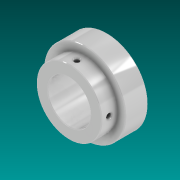
# Autodesk Inventor part: bovenkantGearbox
Saved by Autodesk Inventor 2020.2 (Build 242310000, 310)
## iProperties
Created: 2020-05-14
Part Number: bovenkantGearbox
Material: Aluminum 6061
Document SubType Name: Modeling
Designer: Svend
Density: 2.7 g/cm^3
Appearance: Aluminum - Polished
Author: Svend
Autodesk Inventor part; units mm, degrees
sketch "Sketch1" plane through (0, 0, 0) normal (0, 0, 1) x (1, 0, 0)
  circle A0 centre (0, 0) radius 21
  circle A1 centre (0, 0) radius 12.5
  circle A2 centre (0, 0) radius 11
  point P0 (18, 0)
  point P1 (0, 18)
  point P2 (-18, 0)
  point P3 (0, -18)
  dimension "d0" = 42
  dimension "d1" = 25
  dimension "d2" = 22
  dimension "d3" = 18
  dimension "d6" = 360
  constraints: 6 coincident, 3 centre point, 1 horizontal alignment, 7 other
  measures "d0" diameter of A0
  measures "d1" diameter of A1
  measures "d2" diameter of A2
  measures "d3" distance of A0.centre point (18, 0)
extrude "Extrusion1" add sketch "Sketch1" along normal blind 11.5 contours A0 | A1
extrude "Extrusion2" add sketch "Sketch1" against normal blind 2 contours A1
hole "Hole1" at (18, 0, 0) at (0, 18, 0) at (-18, 0, 0) at (0, -18, 0) direction (0, 0, 1) diameter 3.242 depth 6.5 tip angle 118 countersink diameter 4 countersink angle 90 thread size "M4x0.7" class "6H" standard "ISO Metric profile"
sketch "Sketch2" plane through (0, 0, 11.5) normal (0, 0, 1) x (1, 0, 0)
  circle A0 centre (0, 0) radius 11 projected
  circle A1 centre (0, 0) radius 16.75
  dimension "d19" = 33.5
  constraints: 1 centre point, 1 coincident
  measures "d19" diameter of A1
extrude "Extrusion3" add sketch "Sketch2" along normal blind 8
ref_plane "Work Plane1" through (0, 16.75, 0) normal (0, 1, 0) x (-1, 0, 0)
ref_plane "Work Plane2" through (0, -16.75, 0) normal (0, 1, 0) x (-1, 0, 0)
ref_plane "Work Plane3" through (16.75, 0, 0) normal (1, 0, 0) x (0, 1, 0)
ref_plane "Work Plane4" through (-16.75, 0, 0) normal (1, 0, 0) x (0, 1, 0)
sketch "Sketch3" plane through (-16.75, 0, 0) normal (1, 0, 0) x (0, 1, 0)
  line L0 (21, 11.5) -> (-21, 11.5) projected
  line L1 (16.75, 19.5) -> (-16.75, 19.5) projected
  line L2 (1.621, 0.379) -> (1.621, 6.5) projected
  line L3 (0, 23.4) -> (0, -3.9) projected
  point P0 (0, 0)
  point P1 (0, 15.5)
  dimension "d26" = 4
  constraints: 1 point on line
  measures "d26" distance from line of L1 point (0, 15.5)
sketch "Sketch4" plane through (0, 16.75, 0) normal (0, 1, 0) x (-1, 0, 0)
  line L0 (0, -3.9) -> (0, 23.4) projected
  line L1 (21, 11.5) -> (-21, 11.5) projected
  line L2 (16.75, 19.5) -> (-16.75, 19.5) projected
  point P0 (0, 0)
  point P1 (0, 15.5)
  dimension "d27" = 4
  constraints: 1 point on line
  measures "d27" distance from line of L2 point (0, 15.5)
sketch "Sketch5" plane through (16.75, 0, 0) normal (1, 0, 0) x (0, 1, 0)
  line L0 (0, 23.4) -> (0, -3.9) projected
  line L1 (-16.75, 11.5) -> (16.75, 11.5) projected
  line L2 (16.75, 19.5) -> (-16.75, 19.5) projected
  point P0 (0, 0)
  point P1 (0, 15.5)
  dimension "d28" = 4
  constraints: 1 point on line
  measures "d28" distance from line of L2 point (0, 15.5)
sketch "Sketch6" plane through (0, -16.75, 0) normal (0, 1, 0) x (-1, 0, 0)
  line L0 (0, -3.9) -> (0, 23.4) projected
  line L1 (-16.75, 11.5) -> (16.75, 11.5) projected
  line L2 (16.75, 19.5) -> (-16.75, 19.5) projected
  point P0 (0, 0)
  point P1 (0, 15.5)
  dimension "d29" = 4
  constraints: 1 point on line
  measures "d29" distance from line of L2 point (0, 15.5)
hole "Hole2" at (0, -16.75, 15.5) direction (0, 1, 0) diameter 2.459 depth 5 tip angle 118 countersink diameter 3.5 countersink angle 90 thread size "M3x0.5" class "6H" standard "ISO Metric profile"
hole "Hole3" at (16.75, 0, 15.5) direction (-1, 0, 0) diameter 2.459 depth 5 tip angle 118 countersink diameter 3.5 countersink angle 90 thread size "M3x0.5" class "6H" standard "ISO Metric profile"
hole "Hole4" at (0, 16.75, 15.5) direction (0, -1, 0) diameter 2.459 depth 5 tip angle 118 countersink diameter 3.5 countersink angle 90 thread size "M3x0.5" class "6H" standard "ISO Metric profile"
hole "Hole5" at (-16.75, 0, 15.5) direction (1, 0, 0) diameter 2.459 depth 5 tip angle 118 countersink diameter 3.5 countersink angle 90 thread size "M3x0.5" class "6H" standard "ISO Metric profile"
sketch "Sketch7" plane through (0, 0, 0) normal (0, 0, -1) x (-1, 0, 0)
  circle A0 centre (0, 0) radius 21 projected
  line L0 (-14.8492, -14.8492) -> (14.8492, 14.8492)
  line L1 (21, 0) -> (-21, 0)
  line L2 (-14.8492, 14.8492) -> (14.8492, -14.8492)
  point P0 (-11.3137, 11.3137)
  point P1 (-11.3137, -11.3137)
  point P2 (11.3137, -11.3137)
  point P3 (11.3137, 11.3137)
  dimension "d58" = 45
  dimension "d63" = 16
  dimension "d66" = 360
  constraints: 6 end point, 6 point on circle, 5 midpoint, 1 horizontal, 1 perpendicular, 1 point on line, 5 other
  measures "d58" angle of L0 L1
  measures "d63" distance of point (-11.314, 11.314) point (0, 0)
hole "Hole6" at (11.3137, 11.3137, 0) at (11.3137, -11.3137, 0) at (-11.3137, -11.3137, 0) at (-11.3137, 11.3137, 0) direction (0, 0, 1) diameter 2.459 depth 6.4 tip angle 118 countersink diameter 3.2 countersink angle 90 thread size "M3x0.5" class "6H" standard "ISO Metric profile"
chamfer "Chamfer1" distance 0.3 angle 45 6 edges at (-11, 0, 19.5) (-16.75, 0, 19.5) (-21, 0, 11.5) (-21, 0, 0) (-12.5, 0, -2) (-11, 0, -2)
body "Solid1"
